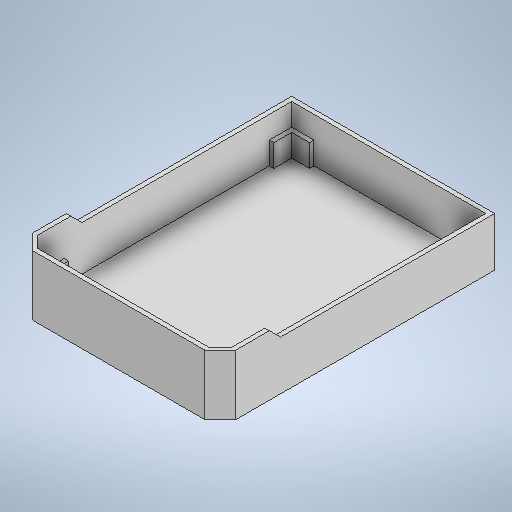
# Autodesk Inventor part: Part1
Saved by Autodesk Inventor 2025.2 (Build 292293000, 293)
## iProperties
Created: 2025-06-04
Part Number: Part1
Material: Generic
Document SubType Name: Sheet Metal
Designer: ziyuz
Density: 1 g/cm^3
Sheet Metal Rule: Default_mm
Appearance: Default
Author: ziyuz
Autodesk Inventor part; units mm, degrees
ref_plane "YZ Plane" through (0, 0, 0) normal (1, 0, 0) x (0, 1, 0)
ref_plane "XZ Plane" through (0, 0, 0) normal (0, 1, 0) x (-1, 0, 0)
ref_plane "XY Plane" through (0, 0, 0) normal (0, 0, 1) x (1, 0, 0)
sketch "Sketch1" plane through (0, 0, 0) normal (0, 1, 0) x (-1, 0, 0)
  line L0 (0, 0) -> (-85, 0)
  line L1 (-85, 0) -> (-85, -115)
  line L2 (-85, -115) -> (0, -115)
  line L3 (0, -115) -> (0, 0)
  dimension "d0" = 85
  dimension "d1" = 115
  constraints: 8 end point, 2 parallel, 1 horizontal, 1 perpendicular
  measures "d0" distance of L2.end L1.end
  measures "d1" distance of L1.end L0.end
extrude "Extrusion1" add sketch "Sketch1" along normal blind 2
sketch "Sketch2" plane through (0, 2, 0) normal (0, 1, 0) x (1, 0, 0)
  line L0 (0, 115) -> (0, 0) projected
  line L1 (0, 115) -> (-2, 115)
  line L2 (0, 115) -> (0, 117)
  line L3 (0, 117) -> (-2, 117)
  line L4 (-2, 115) -> (-2, 117)
  line L5 (-2, 117) -> (87, 117)
  line L6 (87, 117) -> (87, -2)
  line L7 (87, -2) -> (-2, -2)
  line L8 (-2, -2) -> (-2, 117)
  line L9 (-2, 117) -> (-2, 107)
  line L10 (-2, 107) -> (0, 107)
  line L11 (-2, 117) -> (8, 117)
  line L12 (8, 117) -> (8, 115)
  line L13 (85, 115) -> (0, 115) projected
  line L14 (-2, 115) -> (-2, 5)
  line L15 (-2, 5) -> (-2, 15)
  line L16 (0, 15) -> (0, 5)
  line L17 (8, 5) -> (8, 7)
  line L18 (-2, 5) -> (-2, 3)
  line L19 (-2, 3) -> (10, 3)
  line L20 (10, 3) -> (10, 5)
  line L21 (10, 5) -> (0, 5)
  line L22 (0, 5) -> (0, 15)
  line L23 (0, 15) -> (-2, 15)
  line L24 (-2, 5) -> (-2, 15)
  dimension "d4" = 2
  dimension "d5" = 2
  dimension "d6" = 89
  dimension "d7" = 119
  dimension "d8" = 10
  dimension "d9" = 10
  dimension "d10" = 110
  dimension "d11" = 10
  dimension "d13" = 2
  dimension "d21" = 2
  dimension "d22" = 12
  dimension "d23" = 2
  dimension "d24" = 10
  constraints: 46 end point, 9 point on line, 7 perpendicular, 3 parallel, 2 collinear, 2 horizontal, 1 vertical
  measures "d4" distance of L0.start L1.end
  measures "d5" distance of L0.start L2.end
  measures "d6" distance of L6.end L7.end
  measures "d7" distance of L5.end L6.end
  measures "d8" distance of L3.end L9.end
  measures "d9" distance of L3.end L11.end
  measures "d10" distance of L1.end L14.end
  measures "d11" distance of L14.end L15.end
  measures "d13" distance of L17.start L17.end
  measures "d21" distance of L14.end L18.end
  measures "d22" distance of L18.end L19.end
  measures "d23" distance of L19.end L20.end
  measures "d24" distance of L16.end L16.start
extrude "Extrusion2" add sketch "Sketch2" along normal blind 10 contours L0 L10 L8 L1 | L1 L4 L3 L2 | L2 L5 L12 L13 | L0 L19 L8 L23 | L21 L20 L19 L0
sketch "Sketch3" plane through (0, 2, 0) normal (0, -1, 0) x (1, 0, 0)
  line L0 (8, -117) -> (-2, -117) projected
  line L1 (-2, -117) -> (85, -117)
  line L2 (85, -117) -> (85, 2)
  line L3 (85, 2) -> (-2, 2)
  line L4 (-2, 2) -> (-2, -117)
  point P0 (0, 0)
  point P1 (87, -117)
  dimension "d16" = 87
  dimension "d17" = 119
  constraints: 8 end point, 2 parallel, 1 horizontal, 1 perpendicular
  measures "d16" distance of L3.end L2.end
  measures "d17" distance of L2.end L1.end
extrude "Extrusion3" add sketch "Sketch3" along normal blind 2
sketch "Sketch5" plane through (0, 2, 0) normal (0, 1, 0) x (1, 0, 0)
  line L0 (0, 5) -> (0, 15) projected
  line L1 (85, 117) -> (85, -2) projected
  line L2 (0, 5) -> (85, 5)
  line L3 (85, 5) -> (85, 115)
  line L4 (85, 115) -> (0, 115)
  line L5 (0, 115) -> (0, 5)
  line L6 (0, 5) -> (40, 5)
  line L7 (85, 5) -> (50, 5)
  line L8 (85, -2) -> (-2, -2) projected
  line L9 (40, 5) -> (50, 5)
  line L10 (50, 5) -> (50, -2)
  line L11 (50, -2) -> (40, -2)
  line L12 (40, -2) -> (40, 5)
  point P0 (0, 0)
  dimension "d25" = 110
  dimension "d26" = 40
  dimension "d27" = 35
  constraints: 20 end point, 4 parallel, 4 point on line, 2 horizontal, 2 perpendicular
  measures "d25" distance of L3.end L2.end
  measures "d26" distance of L0.start L6.end
  measures "d27" distance of L2.end L7.end
extrude "Extrusion4" cut sketch "Sketch5" against normal blind 10 contours L2 L10 L8 L12
sketch "Sketch6" plane through (0, 0, 0) normal (0, -1, 0) x (1, 0, 0)
  line L0 (-2, 2) -> (-2, -3) projected
  line L1 (-2, 2) -> (-4, 2)
  line L2 (-4, 2) -> (-4, 4)
  line L3 (-4, 4) -> (-2, 4)
  line L4 (-2, 4) -> (-2, 2)
  line L5 (-4, 4) -> (87, 4)
  line L6 (87, 4) -> (87, -119)
  line L7 (87, -119) -> (-4, -119)
  line L8 (-4, -119) -> (-4, 4)
  line L9 (85, -117) -> (85, 2) projected
  line L10 (-2, 2) -> (85, 2)
  line L11 (85, 2) -> (85, -117)
  line L12 (85, -117) -> (-2, -117)
  line L13 (-2, -117) -> (-2, 2)
  line L14 (-2, -3) -> (-4, -3)
  line L15 (-4, -3) -> (-4, 4)
  line L16 (-4, 4) -> (3, 4)
  line L17 (3, 4) -> (3, 2)
  line L18 (-2, -3) -> (3, 2)
  line L19 (85, -3) -> (85, 2)
  line L20 (85, 2) -> (80, 2)
  line L21 (80, 2) -> (85, -3)
  line L22 (87, -3) -> (85, -3)
  line L23 (80, 2) -> (80, 4)
  line L24 (-4, -3) -> (3, 4)
  line L25 (3, 2) -> (-2, -3)
  line L26 (87, -3) -> (80, 4)
  point P0 (0, 0)
  point P1 (85, 2)
  point P2 (-2, -3)
  point P3 (-2, -3)
  dimension "d30" = 2
  dimension "d31" = 2
  dimension "d32" = 91
  dimension "d33" = 123
  dimension "d36" = 7
  dimension "d37" = 5
  constraints: 50 end point, 8 point on line, 7 parallel, 6 perpendicular, 3 horizontal, 2 collinear
  measures "d30" distance of L2.end L3.end
  measures "d31" distance of L1.end L2.end
  measures "d32" distance of L6.end L7.end
  measures "d33" distance of L5.end L6.end
  measures "d36" distance of L2.end L16.end
  measures "d37" distance of L10.end L20.end
extrude "Extrusion5" add sketch "Sketch6" against normal blind 22 contours L24 L10 L18 L0 | L0 L14 L24 | L24 L17 L10 | L13 L12 L9 L22 L6 L7 L8 L14 | L5 L23 L10 L17 | L26 L10 L23 | L10 L26 L9 L21 | L9 L26 L22
sketch "Sketch7" plane through (0, 2, 0) normal (0, 1, 0) x (1, 0, 0)
  line L0 (-2, -2) -> (-2, 1) projected
  line L1 (-2, -2) -> (-2, 1)
  line L2 (1, -2) -> (-2, -2) projected
  line L3 (1, -2) -> (-2, 1)
  line L4 (-2, -2) -> (1, -2)
  line L5 (85, 1) -> (85, -2) projected
  line L6 (85, -2) -> (85, 1)
  line L7 (85, -2) -> (82, -2)
  line L8 (80, -4) -> (87, 3) projected
  line L9 (85, 1) -> (82, -2)
  point P0 (0, 0)
  constraints: 12 end point, 2 collinear, 2 point on line, 2 vertical
extrude "Extrusion6" cut sketch "Sketch7" against normal blind 22
sketch "Sketch8" plane through (0, 22, 0) normal (0, 1, 0) x (1, 0, 0)
  line L0 (-4, 3) -> (-4, 23)
  line L1 (-4, 3) -> (-4, 119) projected
  line L2 (-4, 23) -> (-2, 23)
  line L3 (-2, 3) -> (-2, 117) projected
  line L4 (-2, 3) -> (3, -2) projected
  line L5 (-2, 3) -> (3, -2)
  line L6 (85, 3) -> (80, -2) projected
  line L7 (3, -2) -> (80, -2)
  line L8 (80, -2) -> (85, 3)
  line L9 (85, 117) -> (85, 3) projected
  line L10 (85, 3) -> (85, 23)
  line L11 (85, 23) -> (87, 23)
  line L12 (87, 119) -> (87, 3) projected
  line L13 (80, -4) -> (87, 3) projected
  line L14 (87, 3) -> (87, 23)
  line L15 (87, 3) -> (80, -4)
  line L16 (-4, 3) -> (3, -4) projected
  line L17 (80, -4) -> (3, -4)
  line L18 (3, -4) -> (-4, 3)
  point P0 (0, 0)
  dimension "d40" = 20
  dimension "d41" = 20
  constraints: 22 end point, 5 point on line, 3 collinear, 2 parallel, 2 perpendicular
  measures "d40" distance of L0.start L0.end
  measures "d41" distance of L6.start L10.end
extrude "Extrusion7" add sketch "Sketch8" along normal blind 5
chamfer "Chamfer1" distance 5 angle 45 2 edges at (86, 27, -23) (-3, 27, -23)
equation "\"BendRadius\" = Thickness"
equation "\"BendReliefWidth\" = Thickness"
equation "\"BendReliefDepth\" = 0.5 * Thickness"
equation "\"CornerReliefSize\" = 4 * Thickness"
equation "\"MinimumRemnant\" = 2 * Thickness"
equation "\"TransitionRadius\" = BendRadius"
equation "\"JacobiRadiusSize\" = BendRadius"
equation "\"GapSize\" = Thickness"
equation "\"Thickness\" = 0.5"
body "Solid1"
